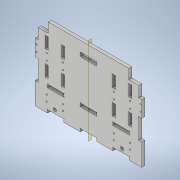
# Autodesk Inventor part: Side_one
Saved by Autodesk Inventor 2020 (Build 240168000, 168)
## iProperties
Created: 2019-12-17
Part Number: Side_one
Material: Generic
Document SubType Name: Modeling
Designer: fabfarm
Density: 1 g/cm^3
Appearance: Default
Author: fabfarm
Autodesk Inventor part; units mm, degrees
ref_plane "YZ Plane" through (0, 0, 0) normal (1, 0, 0) x (0, 1, 0)
ref_plane "XZ Plane" through (0, 0, 0) normal (0, 1, 0) x (-1, 0, 0)
ref_plane "XY Plane" through (0, 0, 0) normal (0, 0, 1) x (1, 0, 0)
sketch "Sketch1" plane through (0, 0, 0) normal (0, 0, 1) x (1, 0, 0)
  line L0 (0, 0) -> (-652, 0)
  line L1 (-652, 0) -> (-652, 485)
  line L2 (-652, 485) -> (0, 485)
  line L3 (0, 485) -> (0, 0)
  dimension "d0" = 485
  dimension "d1" = 652
  constraints: 8 end point, 2 parallel, 1 horizontal, 1 perpendicular
  measures "d0" distance of L2.end L0.start
  measures "d1" distance of L0.start L0.end
extrude "Extrusion1" add sketch "Sketch1" along normal blind 18.55
sketch "Sketch2" plane through (0, 0, 18.55) normal (0, 0, 1) x (1, 0, 0)
  line L0 (-652, 485) -> (-652, 0) projected
  line L1 (-652, 485) -> (-633.45, 485)
  line L2 (-633.45, 485) -> (-633.45, 359.9)
  line L3 (-633.45, 359.9) -> (-652, 359.9)
  line L4 (-652, 359.9) -> (-652, 485)
  line L5 (0, 485) -> (-652, 485) projected
  line L6 (-652, 259.9) -> (-633.45, 259.9)
  line L7 (-633.45, 259.9) -> (-633.45, 134.8)
  line L8 (-633.45, 134.8) -> (-652, 134.8)
  line L9 (-652, 134.8) -> (-652, 259.9)
  point P0 (-652, 359.9)
  dimension "d54" = 18.55
  dimension "d55" = 125.1
  dimension "d86" = 100
  dimension "d87" = 125.1
  constraints: 16 end point, 4 parallel, 2 collinear, 2 horizontal, 2 perpendicular, 2 point on line
  measures "d54" distance of L1.start L1.end
  measures "d55" distance of L1.end L2.end
  measures "d86" distance between parallel lines of L6 L3
  measures "d87" distance of L6.end L7.end
extrude "Extrusion2" cut sketch "Sketch2" against normal blind 18.55
ref_plane "Work Plane1" through (-326, 259.9, 0) normal (-1, 0, 0) x (0, 0, 1)
mirror "Mirror1" about plane through (-326, 259.9, 0) normal (-1, 0, 0) of "Extrusion2"
sketch "Sketch3" plane through (0, 0, 18.55) normal (0, 0, 1) x (1, 0, 0)
  line L0 (0, 485) -> (-652, 485) projected
  line L1 (-652, 425) -> (-572, 425)
  line L2 (-572, 425) -> (-572, 485)
  line L3 (-572, 485) -> (-652, 485)
  line L4 (-652, 485) -> (-652, 425)
  point P0 (0, 0)
  point P1 (-18.55, 350)
  point P2 (0, 485)
  dimension "d19" = 80
  dimension "d22" = 60
  constraints: 8 end point, 2 perpendicular, 1 parallel, 2 other
  measures "d19" distance of L3.end L2.end
  measures "d22" distance of L3.end L1.start
extrude "Extrusion3" cut sketch "Sketch3" against normal blind 18.55
mirror "Mirror2" about plane through (-326, 259.9, 0) normal (-1, 0, 0) of "Extrusion3"
sketch "Sketch4" plane through (0, 0, 18.55) normal (0, 0, 1) x (1, 0, 0)
  line L0 (-576.1, 134.8) -> (-475.9, 134.8)
  line L1 (-475.9, 134.8) -> (-475.9, 153.45)
  line L2 (-475.9, 153.45) -> (-576.1, 153.45)
  line L3 (-576.1, 153.45) -> (-576.1, 134.8)
  line L4 (-376.1, 134.8) -> (-275.9, 134.8)
  line L5 (-275.9, 134.8) -> (-275.9, 153.45)
  line L6 (-275.9, 153.45) -> (-376.1, 153.45)
  line L7 (-376.1, 153.45) -> (-376.1, 134.8)
  line L8 (-176.1, 134.8) -> (-75.9, 134.8)
  line L9 (-75.9, 134.8) -> (-75.9, 153.45)
  line L10 (-75.9, 153.45) -> (-176.1, 153.45)
  line L11 (-176.1, 153.45) -> (-176.1, 134.8)
  line L12 (0, 0) -> (0, 359.9) projected
  line L13 (-652, 359.9) -> (-652, 0) projected
  line L14 (-633.45, 134.8) -> (-652, 134.8) projected
  line L15 (-652, 259.9) -> (-633.45, 259.9) projected
  dimension "d59" = 100.2
  dimension "d60" = 100.2
  dimension "d61" = 99.8
  dimension "d62" = 99.8
  dimension "d63" = 100.2
  dimension "d66" = 18.65
  dimension "d67" = 75.9
  constraints: 24 end point, 6 parallel, 5 collinear, 3 horizontal, 3 perpendicular
  measures "d59" distance of L1.end L2.end
  measures "d60" distance of L5.end L6.end
  measures "d61" distance between parallel lines of L1 L7
  measures "d62" distance between parallel lines of L11 L5
  measures "d63" distance of L9.end L10.end
  measures "d66" distance of L2.end L0.start
  measures "d67" distance between parallel lines of L12 L9
extrude "Extrusion4" cut sketch "Sketch4" against normal blind 20
sketch "Sketch6" plane through (0, 0, 18.55) normal (0, 0, 1) x (1, 0, 0)
  line L0 (-276, 400) -> (-376, 400)
  line L1 (-376, 400) -> (-376, 425)
  line L2 (-376, 425) -> (-276, 425)
  line L3 (-276, 425) -> (-276, 400)
  line L4 (-276, 400) -> (-376, 425) construction
  line L5 (-376, 400) -> (-276, 425) construction
  line L6 (-326, -97) -> (-326, 582) projected
  line L7 (-80, 485) -> (-572, 485) projected
  point P0 (0, 0)
  point P1 (-326, 412.5)
  dimension "d38" = 25
  dimension "d39" = 100
  dimension "d40" = 60
  constraints: 12 end point, 2 midpoint, 2 parallel, 1 horizontal, 1 perpendicular, 1 point on line
  measures "d38" distance of L0.end L1.end
  measures "d39" distance of L1.end L2.end
  measures "d40" distance between parallel lines of L7 L2
extrude "Extrusion6" cut sketch "Sketch6" against normal blind 20
fillet "Fillet1" radius 4 4 edges at (-276, 425, 9.275) (-276, 400, 9.275) (-376, 425, 9.275) (-376, 400, 9.275)
sketch "Sketch7" plane through (0, 0, 18.55) normal (0, 0, 1) x (1, 0, 0)
  line L0 (-590.85, 183.95) -> (-572, 183.95)
  line L1 (-572, 183.95) -> (-572, 254.45)
  line L2 (-572, 254.45) -> (-590.85, 254.45)
  line L3 (-590.85, 254.45) -> (-590.85, 183.95)
  line L4 (-491, 183.95) -> (-472.15, 183.95)
  line L5 (-472.15, 183.95) -> (-472.15, 254.45)
  line L6 (-472.15, 254.45) -> (-491, 254.45)
  line L7 (-491, 254.45) -> (-491, 183.95)
  line L8 (-572, 485) -> (-572, 425) projected
  line L9 (-576.1, 153.45) -> (-475.9, 153.45) projected
  point P0 (0, 0)
  point P1 (-572, 290)
  dimension "d44" = 81
  dimension "d45" = 18.85
  dimension "d46" = 70.5
  dimension "d72" = 30.5
  constraints: 16 end point, 4 parallel, 2 collinear, 2 horizontal, 2 perpendicular, 2 point on line
  measures "d44" distance between parallel lines of L7 L1
  measures "d45" distance of L1.end L2.end
  measures "d46" distance of L2.end L0.start
  measures "d72" distance between parallel lines of L9 L0
extrude "Extrusion7" cut sketch "Sketch7" against normal blind 20
mirror "Mirror3" about plane through (-326, 259.9, 0) normal (-1, 0, 0) of "Extrusion7"
sketch "Esquisse8" plane through (0, 0, 0) normal (0, 0, -1) x (-1, 0, 0)
  line L0 (80, 334.95) -> (61.15, 334.95)
  line L1 (61.15, 334.95) -> (61.15, 405.45)
  line L2 (61.15, 405.45) -> (80, 405.45)
  line L3 (80, 405.45) -> (80, 334.95)
  line L4 (161, 405.45) -> (179.85, 405.45)
  line L5 (179.85, 405.45) -> (179.85, 334.95)
  line L6 (179.85, 334.95) -> (161, 334.95)
  line L7 (161, 334.95) -> (161, 405.45)
  line L8 (61.15, 183.95) -> (61.15, 254.45) projected
  line L9 (80, 254.45) -> (80, 183.95) projected
  line L10 (161, 183.95) -> (161, 254.45) projected
  line L11 (179.85, 254.45) -> (179.85, 183.95) projected
  line L12 (80, 254.45) -> (61.15, 254.45) projected
  point P0 (0, 0)
  dimension "d51" = 70.5
  dimension "d90" = 80.5
  constraints: 16 end point, 4 collinear, 4 parallel, 2 horizontal, 2 perpendicular, 2 point on line
  measures "d51" distance of L0.end L1.end
  measures "d90" distance between parallel lines of L0 L12
extrude "Extrusion8" cut sketch "Esquisse8" against normal blind 20
mirror "Symétrie4" about plane through (-326, 259.9, 0) normal (-1, 0, 0) of "Extrusion8"
sketch "Esquisse9" plane through (0, 0, 18.55) normal (0, 0, 1) x (1, 0, 0)
  line L0 (-652, 359.9) -> (-633.45, 359.9) construction
  circle A0 centre (-633.45, 359.9) radius 1.585
  circle A1 centre (-633.45, 134.8) radius 1.585
  line L1 (-572, 183.95) -> (-572, 405.45) construction
  circle A2 centre (-572, 405.45) radius 1.585
  line L2 (-590.85, 405.45) -> (-572, 405.45) construction
  circle A3 centre (-590.85, 405.45) radius 1.585
  circle A4 centre (-590.85, 334.95) radius 1.585
  circle A5 centre (-633.45, 259.9) radius 1.585
  line L3 (-590.85, 254.45) -> (-572, 254.45) construction
  circle A6 centre (-590.85, 254.45) radius 1.585
  circle A7 centre (-572, 254.45) radius 1.585
  circle A8 centre (-590.85, 183.95) radius 1.585
  line L4 (-572, 183.95) -> (-590.85, 183.95) construction
  circle A9 centre (-572, 183.95) radius 1.585
  line L5 (-633.45, 425) -> (-572, 425) construction
  circle A10 centre (-572, 425) radius 1.585
  line L6 (-576.1, 153.45) -> (-475.9, 153.45) construction
  circle A11 centre (-576.1, 153.45) radius 1.585
  circle A12 centre (-475.9, 153.45) radius 1.585
  line L7 (-491, 183.95) -> (-472.15, 183.95) construction
  circle A13 centre (-491, 183.95) radius 1.585
  circle A14 centre (-472.15, 183.95) radius 1.585
  circle A15 centre (-491, 254.45) radius 1.585
  circle A16 centre (-472.15, 254.45) radius 1.585
  line L8 (-376.1, 153.45) -> (-275.9, 153.45) construction
  circle A17 centre (-376.1, 153.45) radius 1.585
  circle A18 centre (-491, 405.45) radius 1.585
  circle A19 centre (-472.15, 405.45) radius 1.585
  circle A20 centre (-491, 334.95) radius 1.585
  circle A21 centre (-472.15, 334.95) radius 1.585
  line L9 (-590.85, 183.95) -> (-590.85, 254.45) construction
  line L10 (-491, 405.45) -> (-472.15, 405.45) construction
  line L11 (-491, 183.95) -> (-491, 405.45) construction
  line L12 (-572, 485) -> (-80, 485) projected
  line L13 (-326, 485) -> (-326, 153.45) construction
  line L14 (-572, 254.45) -> (-572, 183.95) projected
  line L15 (-472.15, 405.45) -> (-472.15, 183.95) construction
  line L16 (-472.15, 334.95) -> (-491, 334.95) projected
  circle A22 centre (-576.1, 134.8) radius 1.585
  line L17 (-475.9, 153.45) -> (-475.9, 134.8) projected
  circle A23 centre (-475.9, 134.8) radius 1.585
  line L18 (-376.1, 134.8) -> (-376.1, 153.45) projected
  circle A24 centre (-376.1, 134.8) radius 1.585
  line L19 (0, 359.9) -> (-18.55, 359.9) construction
  circle A25 centre (-18.55, 359.9) radius 1.585
  circle A26 centre (-18.55, 134.8) radius 1.585
  line L20 (-80, 183.95) -> (-80, 405.45) construction
  circle A27 centre (-80, 405.45) radius 1.585
  line L21 (-61.15, 405.45) -> (-80, 405.45) construction
  circle A28 centre (-61.15, 405.45) radius 1.585
  circle A29 centre (-61.15, 334.95) radius 1.585
  circle A30 centre (-18.55, 259.9) radius 1.585
  line L22 (-61.15, 254.45) -> (-80, 254.45) construction
  circle A31 centre (-61.15, 254.45) radius 1.585
  circle A32 centre (-80, 254.45) radius 1.585
  circle A33 centre (-61.15, 183.95) radius 1.585
  line L23 (-80, 183.95) -> (-61.15, 183.95) construction
  circle A34 centre (-80, 183.95) radius 1.585
  line L24 (-18.55, 425) -> (-80, 425) construction
  circle A35 centre (-80, 425) radius 1.585
  line L25 (-75.9, 153.45) -> (-176.1, 153.45) construction
  circle A36 centre (-75.9, 153.45) radius 1.585
  circle A37 centre (-176.1, 153.45) radius 1.585
  line L26 (-161, 183.95) -> (-179.85, 183.95) construction
  circle A38 centre (-161, 183.95) radius 1.585
  circle A39 centre (-179.85, 183.95) radius 1.585
  circle A40 centre (-161, 254.45) radius 1.585
  circle A41 centre (-179.85, 254.45) radius 1.585
  circle A42 centre (-275.9, 153.45) radius 1.585
  circle A43 centre (-161, 405.45) radius 1.585
  circle A44 centre (-179.85, 405.45) radius 1.585
  circle A45 centre (-161, 334.95) radius 1.585
  circle A46 centre (-179.85, 334.95) radius 1.585
  line L27 (-61.15, 183.95) -> (-61.15, 254.45) construction
  line L28 (-161, 405.45) -> (-179.85, 405.45) construction
  line L29 (-161, 183.95) -> (-161, 405.45) construction
  line L30 (-80, 254.45) -> (-80, 183.95)
  line L31 (-179.85, 405.45) -> (-179.85, 183.95) construction
  line L32 (-179.85, 334.95) -> (-161, 334.95)
  circle A47 centre (-75.9, 134.8) radius 1.585
  line L33 (-176.1, 153.45) -> (-176.1, 134.8)
  circle A48 centre (-176.1, 134.8) radius 1.585
  line L34 (-275.9, 134.8) -> (-275.9, 153.45)
  circle A49 centre (-275.9, 134.8) radius 1.585
  point P0 (-572, 334.95)
  point P1 (-80, 334.95)
  dimension "d69" = 3.17
  constraints: 50 centre point, 40 symmetric about line, 34 end point, 24 equal radius, 16 point on line, 14 coincident, 2 midpoint, 25 other
  measures "d69" diameter of A7
extrude "Extrusion9" cut sketch "Esquisse9" against normal blind 20 contours A11 | A12 | A17 | A22 | A23 | A24 | A25 | A26 | A27 | A28 | A29 | A30 | A31 | A32 | A33 | A34 | A35 | A36 | A37 | A38 | A39 | A40 | A41 | A42 | A43 | A44 | A45 | A46 | A47 | A48 | A49
sketch "Esquisse11" plane through (0, 0, 18.55) normal (0, 0, 1) x (1, 0, 0)
  circle A0 centre (-643.5175, 329.9) radius 4
  circle A1 centre (-643.5175, 289.9) radius 4
  circle A2 centre (-580.8314, 314.95) radius 4
  circle A3 centre (-581.2288, 274.45) radius 4
  circle A4 centre (-481.575, 314.95) radius 4
  circle A5 centre (-481.575, 274.45) radius 4
  line L0 (-572, 334.95) -> (-590.85, 334.95) projected
  line L1 (-580.6351, 334.95) -> (-581.425, 254.45) construction
  line L2 (-590.85, 254.45) -> (-572, 254.45) projected
  line L3 (-472.15, 334.95) -> (-491, 334.95) projected
  line L4 (-481.575, 334.95) -> (-481.575, 254.45) construction
  line L5 (-491, 254.45) -> (-472.15, 254.45) projected
  line L6 (-633.45, 359.9) -> (-652, 359.9) projected
  line L7 (-80, 485) -> (-572, 485) projected
  line L8 (-326, 485) -> (-325.2075, 153.45) construction
  line L9 (-376.1, 153.45) -> (-275.9, 153.45) projected
  circle A6 centre (-7.7447, 331.4197) radius 4
  circle A7 centre (-7.5534, 291.4201) radius 4
  circle A8 centre (-70.3586, 316.1702) radius 4
  circle A9 centre (-69.7676, 275.6725) radius 4
  circle A10 centre (-169.6138, 315.6957) radius 4
  circle A11 centre (-169.4202, 275.1961) radius 4
  line L10 (-70.6505, 336.169) -> (-69.4758, 255.6737) construction
  line L11 (-61.632, 254.9112) -> (-77.3118, 254.8362)
  line L12 (-177.5479, 335.358) -> (-161.8681, 335.4329)
  line L13 (-169.7095, 335.6954) -> (-169.3246, 255.1964) construction
  line L14 (-161.4809, 254.4339) -> (-177.1607, 254.3589)
  line L15 (-16.3705, 361.3788) -> (0.5943, 361.4599)
  line L16 (-652, 259.9) -> (-633.45, 259.9) projected
  line L17 (-643.5175, 359.9) -> (-643.5175, 259.9) construction
  point P0 (-573.5723, 199.8)
  point P1 (-589.265, 334.65)
  point P2 (-589.265, 253.65)
  point P3 (-573.585, 253.65)
  point P4 (-473.735, 334.65)
  point P5 (-489.415, 334.65)
  point P6 (-489.415, 253.65)
  point P7 (-473.735, 253.65)
  point P8 (-635.035, 359.9)
  point P9 (-374.515, 153.45)
  point P10 (-277.485, 153.35)
  point P11 (-61.632, 254.9112)
  point P12 (-77.3118, 254.8362)
  point P13 (-177.5479, 335.358)
  point P14 (-161.8681, 335.4329)
  point P15 (-161.4809, 254.4339)
  point P16 (-177.1607, 254.3589)
  point P17 (-275.9, 153.45)
  point P18 (-635.035, 259.9)
  dimension "d76" = 8
  dimension "d79" = 30
  dimension "d80" = 20
  dimension "d81" = 20
  dimension "d82" = 20
  dimension "d83" = 20
  dimension "d91" = 30
  constraints: 18 symmetric about line, 14 end point, 12 centre point, 12 point on line, 5 equal radius, 1 midpoint, 25 other
  measures "d76" diameter of A0
  measures "d79" distance from line of L6 A0.centre
  measures "d91" distance from line of A1.centre L16
extrude "Extrusion10" cut sketch "Esquisse11" against normal blind 20
sketch "Esquisse12" plane through (0, 0, 18.55) normal (0, 0, 1) x (1, 0, 0)
  line L0 (0, 0) -> (-652, 0) projected
  line L1 (-576.1, 0) -> (-475.9, 0)
  line L2 (-475.9, 0) -> (-475.9, 18.55)
  line L3 (-475.9, 18.55) -> (-576.1, 18.55)
  line L4 (-576.1, 18.55) -> (-576.1, 0)
  line L5 (-376.1, 0) -> (-275.9, 0)
  line L6 (-275.9, 0) -> (-275.9, 18.55)
  line L7 (-275.9, 18.55) -> (-376.1, 18.55)
  line L8 (-376.1, 18.55) -> (-376.1, 0)
  line L9 (-176.1, 0) -> (-75.9, 0)
  line L10 (-75.9, 0) -> (-75.9, 18.55)
  line L11 (-75.9, 18.55) -> (-176.1, 18.55)
  line L12 (-176.1, 18.55) -> (-176.1, 0)
  line L13 (-475.9, 151.865) -> (-475.9, 136.385) projected
  line L14 (-576.1, 136.385) -> (-576.1, 151.865) projected
  line L15 (-376.1, 136.385) -> (-376.1, 151.865) projected
  line L16 (-275.9, 151.865) -> (-275.9, 136.385) projected
  line L17 (-176.1, 136.385) -> (-176.1, 151.865) projected
  line L18 (-75.9, 151.865) -> (-75.9, 136.385) projected
  point P0 (-75.9, 0)
  dimension "d92" = 18.55
  constraints: 24 end point, 7 collinear, 6 parallel, 4 point on line, 3 horizontal, 3 perpendicular
  measures "d92" distance of L3.end L1.start
extrude "Extrusion11" cut sketch "Esquisse12" against normal blind 20
sketch "Esquisse13" plane through (0, 0, 18.55) normal (0, 0, 1) x (1, 0, 0)
  line L0 (-576.1, 18.55) -> (-576.1, 0) projected
  circle A0 centre (-576.1, 18.55) radius 1.6
  line L1 (-475.9, 18.55) -> (-576.1, 18.55) projected
  circle A1 centre (-475.9, 18.55) radius 1.6
  line L2 (-376.1, 18.55) -> (-275.9, 18.55) projected
  circle A2 centre (-376.1, 18.55) radius 1.6
  circle A3 centre (-275.9, 18.55) radius 1.6
  circle A4 centre (-176.1, 18.55) radius 1.6
  line L3 (-75.9, 18.55) -> (-176.1, 18.55) projected
  circle A5 centre (-75.9, 18.55) radius 1.6
  point P0 (0, 0)
  dimension "d95" = 3.2
  constraints: 6 centre point, 5 equal radius, 1 coincident
  measures "d95" diameter of A0
extrude "Extrusion12" cut sketch "Esquisse13" against normal blind 20
sketch "Esquisse14" plane through (0, 0, 18.55) normal (0, 0, 1) x (1, 0, 0)
  circle A0 centre (-581.425, 94.8) radius 4
  circle A1 centre (-581.425, 58.55) radius 4
  circle A2 centre (-481.575, 94.8) radius 4
  circle A3 centre (-481.575, 58.55) radius 4
  line L0 (-572, 183.95) -> (-590.85, 183.95) projected
  line L1 (-581.425, 183.95) -> (-581.425, 0) construction
  line L2 (-576.1, 0) -> (-652, 0) projected
  line L3 (-472.15, 183.95) -> (-491, 183.95) projected
  line L4 (-481.575, 183.95) -> (-481.575, 0.5) construction
  line L5 (-574.5, 18.55) -> (-477.5, 18.55) projected
  line L6 (-477.485, 134.8) -> (-574.515, 134.8) projected
  line L7 (-374.5, 18.55) -> (-277.5, 18.55) projected
  line L8 (-326, 18.55) -> (-326, 134.8) construction
  line L9 (-277.485, 134.8) -> (-374.515, 134.8) projected
  circle A4 centre (-70.575, 94.8) radius 4
  circle A5 centre (-70.575, 58.55) radius 4
  circle A6 centre (-170.425, 94.8) radius 4
  circle A7 centre (-170.425, 58.55) radius 4
  point P0 (0, 0)
  dimension "d98" = 8
  dimension "d99" = 40
  dimension "d100" = 40
  dimension "d101" = 40
  dimension "d103" = 40
  constraints: 8 centre point, 6 end point, 5 point on line, 4 midpoint, 4 symmetric about line, 3 equal radius, 2 vertical, 4 other
  measures "d98" diameter of A0
  measures "d99" distance from line of L5 A3.centre
  measures "d100" distance from line of L6 A2.centre
  measures "d101" distance from line of L6 A0.centre
  measures "d103" distance from line of L5 A1.centre
extrude "Extrusion13" cut sketch "Esquisse14" against normal blind 20
sketch "Esquisse15" plane through (0, 0, 18.55) normal (0, 0, 1) x (1, 0, 0)
  circle A0 centre (-531.5, 39.8) radius 10
  line L0 (-574.5, 18.55) -> (-477.5, 18.55) projected
  line L1 (-477.5, 18.55) -> (-574.5, 18.55) projected
  line L2 (-572, 183.95) -> (-572, 254.45) projected
  line L3 (-572, 219.2) -> (-491, 219.2) construction
  line L4 (-491, 254.45) -> (-491, 183.95) projected
  line L5 (-531.5, 219.2) -> (-531.5, 18.55) construction
  line L6 (-374.515, 134.8) -> (-277.485, 134.8) projected
  line L7 (-326, 134.8) -> (-326, 18.55) construction
  circle A1 centre (-120.5, 39.8) radius 10
  point P0 (0, 0)
  dimension "d106" = 21.25
  dimension "d107" = 20
  constraints: 6 end point, 4 midpoint, 2 centre point, 2 point on line, 1 perpendicular, 1 symmetric about line, 1 vertical, 1 other
  measures "d106" distance from line of L0 A0.centre
  measures "d107" diameter of A0
extrude "Extrusion14" cut sketch "Esquisse15" against normal blind 20
body "Solid1"
